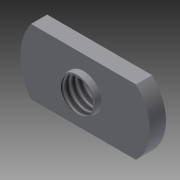
# Autodesk Inventor part: 3786_economy_slide_tnuts
Saved by Autodesk Inventor 2014 (Build 180170000, 170)
## iProperties
Created: 2014-10-05
Part Number: 3786_economy_slide_tnuts
Material: Generic
Document SubType Name: Modeling
Designer: Matthew
Density: 1 g/cm^3
Appearance: Default
Author: Matthew
Autodesk Inventor part; units mm, degrees
ref_plane "YZ Plane" through (0, 0, 0) normal (1, 0, 0) x (0, 1, 0)
ref_plane "XZ Plane" through (0, 0, 0) normal (0, 1, 0) x (-1, 0, 0)
ref_plane "XY Plane" through (0, 0, 0) normal (0, 0, 1) x (1, 0, 0)
sketch "Sketch1" plane through (0, 0, 0) normal (0, 0, 1) x (1, 0, 0)
  line L0 (-10.3124, -6.4135) -> (10.3124, -6.4135)
  line L1 (10.3124, -6.4135) -> (10.3124, 6.4135) construction
  line L2 (10.3124, 6.4135) -> (-10.3124, 6.4135)
  line L3 (-10.3124, 6.4135) -> (-10.3124, -6.4135) construction
  line L4 (-10.3124, -6.4135) -> (10.3124, 6.4135) construction
  line L5 (10.3124, -6.4135) -> (-10.3124, 6.4135) construction
  arc A0 (10.3124, -6.4135) -> (10.3124, 6.4135) centre (4.1562, 0) ccw
  arc A1 (-10.3124, 6.4135) -> (-10.3124, -6.4135) centre (-1.4224, 0) ccw
  point P0 (0, 0)
  dimension "d0" = 12.827
  dimension "d1" = 8.89
  dimension "d2" = 8.89
  dimension "d3" = 1.4224
  constraints: 12 end point, 4 point on circle, 2 centre point, 2 midpoint, 2 parallel, 1 horizontal, 1 perpendicular
  measures "d0" distance between parallel lines of L0 L2
  measures "d1" radius of A0
  measures "d2" distance from line of L3 A1.centre
  measures "d3" distance of point (0, 0) A1.centre
extrude "Extrusion1" add sketch "Sketch1" along normal blind 3.175
sketch "Sketch2" plane through (0, 0, 0) normal (0, 0, -1) x (-1, 0, 0)
  circle A0 centre (0, 0) radius 3.175
  dimension "d6" = 6.35
  constraints: 1 centre point, 1 coincident
  measures "d6" diameter of A0
extrude "Extrusion2" cut sketch "Sketch2" against normal blind 5.08
sketch "Sketch3" plane through (0, 0, 3.175) normal (0, 0, 1) x (1, 0, 0)
  circle A0 centre (0, 0) radius 3.175 projected
  circle A1 centre (0, 0) radius 3.556
  dimension "d9" = 7.112
  constraints: 1 centre point, 1 coincident
  measures "d9" diameter of A1
extrude "Extrusion3" add sketch "Sketch3" along normal blind 1.27
thread "Thread1" size "1/4-20 UNC" class "2B" standard "ANSI Unified Screw Threads" full length
equation "\"d2\" = d1"
body "Solid1"
